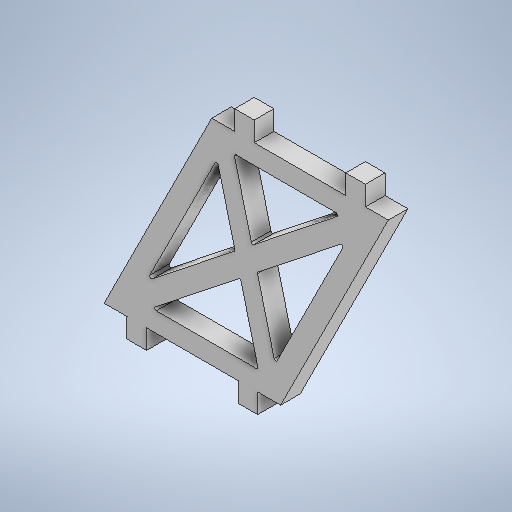
# Autodesk Inventor part: ENTRE_ASA
Saved by Autodesk Inventor 2025.1 (Build 291241000, 241)
## iProperties
Created: 2024-10-24
Part Number: ENTRE_ASA
Material: Genérico
Document SubType Name: Modeling
Designer: ambrosildo
Density: 1 g/cm^3
Appearance: Padrão
Author: ambrosildo
Autodesk Inventor part; units mm, degrees
ref_plane "YZ Plane" through (0, 0, 0) normal (1, 0, 0) x (0, 1, 0)
ref_plane "XZ Plane" through (0, 0, 0) normal (0, 1, 0) x (-1, 0, 0)
ref_plane "XY Plane" through (0, 0, 0) normal (0, 0, 1) x (1, 0, 0)
sketch "Esboço1" plane through (0, 0, 0) normal (0, 0, 1) x (1, 0, 0)
  line L0 (0, 0) -> (16.4719, 32.7528)
  line L1 (16.4719, 32.7528) -> (43.4719, 32.7528)
  line L2 (0, 0) -> (27, 0)
  line L3 (27, 0) -> (43.4719, 32.7528)
  line L4 (16.9941, 27.1139) -> (6.9771, 7.1962)
  line L5 (35.4733, 29.7528) -> (20.1912, 29.7528)
  line L6 (23.2808, 3) -> (7.9986, 3)
  line L7 (36.4948, 25.5566) -> (26.4779, 5.6389)
  arc A0 (7.8433, 3.4459) -> (7.9986, 3) centre (7.9986, 3.25) ccw
  arc A1 (6.9771, 7.1962) -> (7.3558, 6.888) centre (7.2005, 7.0839) ccw
  arc A2 (36.4948, 25.5566) -> (36.1161, 25.8648) centre (36.2715, 25.6689) ccw
  arc A3 (35.6286, 29.3069) -> (35.4733, 29.7528) centre (35.4733, 29.5028) ccw
  arc A4 (17.4597, 27.0634) -> (16.9941, 27.1139) centre (17.2174, 27.0016) ccw
  arc A5 (20.1912, 29.7528) -> (19.9489, 29.441) centre (20.1912, 29.5028) ccw
  line L8 (17.4597, 27.0634) -> (20.002, 17.1046)
  line L9 (20.9503, 13.3898) -> (23.523, 3.3118)
  line L10 (36.1161, 25.8648) -> (23.5569, 15.9059)
  line L11 (20.5527, 13.5238) -> (7.8433, 3.4459)
  line L12 (19.9489, 29.441) -> (22.5216, 19.363)
  line L13 (23.47, 15.6482) -> (26.0123, 5.6894)
  line L14 (35.6286, 29.3069) -> (22.9192, 19.229)
  line L15 (19.9151, 16.8469) -> (7.3558, 6.888)
  arc A6 (20.9503, 13.3898) -> (20.5527, 13.5238) centre (20.7081, 13.3279) ccw
  arc A7 (19.9151, 16.8469) -> (20.002, 17.1046) centre (19.7597, 17.0428) ccw
  arc A8 (22.5216, 19.363) -> (22.9192, 19.229) centre (22.7639, 19.4249) ccw
  arc A9 (23.5569, 15.9059) -> (23.47, 15.6482) centre (23.7122, 15.71) ccw
  arc A10 (23.2808, 3) -> (23.523, 3.3118) centre (23.2808, 3.25) ccw
  arc A11 (26.0123, 5.6894) -> (26.4779, 5.6389) centre (26.2545, 5.7512) ccw
  constraints: 32 end point, 30 tangent, 24 point on circle, 12 centre point, 7 horizontal, 12 other
extrude "Extrusão1" add sketch "Esboço1" along normal blind 3
sketch "Esboço2" plane through (16.4719, 32.7528, 0) normal (0, 1, 0) x (1, 0, 0)
  line L0 (27, 0) -> (0, 0) projected
  line L1 (27, -3) -> (0, -3) projected
  line L2 (23.5, 0) -> (20.5, 0)
  line L3 (20.5, 0) -> (20.5, -3)
  line L4 (20.5, -3) -> (23.5, -3)
  line L5 (23.5, -3) -> (23.5, 0)
  line L6 (3.5, 0) -> (6.5, 0)
  line L7 (6.5, 0) -> (6.5, -3)
  line L8 (6.5, -3) -> (3.5, -3)
  line L9 (3.5, -3) -> (3.5, 0)
  point P0 (-16.4719, 0)
  point P1 (3.5, -3)
  point P2 (6.5, -3)
  point P3 (6.5, 0)
  dimension "d13" = 3
  dimension "d14" = 3
  dimension "d61" = 3
  dimension "d62" = 3
  constraints: 16 end point, 4 parallel, 2 horizontal, 2 perpendicular, 2 point on line
  measures "d13" distance of L4.end L3.end
  measures "d14" distance of L3.end L2.end
  measures "d61" distance of L7.end L8.end
  measures "d62" distance of L6.end L7.end
extrude "Extrusão2" add sketch "Esboço2" along normal blind 3 contours L5 L1 L3 L0 | L7 L1 L9 L0
sketch "Esboço3" plane through (0, 0, 0) normal (0, -1, 0) x (1, 0, 0)
  line L0 (3.5, 3) -> (6.5, 3)
  line L1 (6.5, 3) -> (6.5, 0)
  line L2 (6.5, 0) -> (3.5, 0)
  line L3 (3.5, 0) -> (3.5, 3)
  line L4 (23.4939, 3) -> (20.4939, 3)
  line L5 (20.4939, 3) -> (20.4939, 0)
  line L6 (20.4939, 0) -> (23.4939, 0)
  line L7 (23.4939, 0) -> (23.4939, 3)
  point P0 (0, 0)
  dimension "d65" = 3
  dimension "d66" = 3
  dimension "d67" = 3
  dimension "d68" = 3
  constraints: 16 end point, 4 parallel, 2 horizontal, 2 perpendicular
  measures "d65" distance of L1.end L2.end
  measures "d66" distance of L0.end L1.end
  measures "d67" distance of L6.end L5.end
  measures "d68" distance of L5.end L4.end
extrude "Extrusão3" add sketch "Esboço3" along normal blind 3
